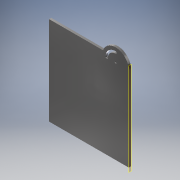
# Autodesk Inventor part: Base
Saved by Autodesk Inventor 2018 (Build 220112000, 112)
## iProperties
Created: 2021-07-05
Part Number: Base
Material: Acero, fundido
Document SubType Name: Modeling
Designer: GABRIEL
Density: 7.85 g/cm^3
Appearance: Semipulido
Author: GABRIEL
Autodesk Inventor part; units mm, degrees
ref_plane "YZ Plane" through (0, 0, 0) normal (1, 0, 0) x (0, 1, 0)
ref_plane "XZ Plane" through (0, 0, 0) normal (0, 1, 0) x (-1, 0, 0)
ref_plane "XY Plane" through (0, 0, 0) normal (0, 0, 1) x (1, 0, 0)
sketch "Boceto2" plane through (0, 0, 0) normal (0, 1, 0) x (-1, 0, 0)
  line L0 (-420, -20) -> (-420, -400)
  line L1 (-420, -400) -> (-60, -400)
  line L2 (-60, -400) -> (-60, 0)
  line L3 (-60, 0) -> (-303.4315, 0)
  arc A0 (-303.4315, 0) -> (-420, -20) centre (-360, -20) ccw
  circle A1 centre (-360, -20) radius 4
  circle A2 centre (-360, 20) radius 5
  circle A3 centre (-320, -20) radius 5
  arc A4 (-325, -20) -> (-360, 15) centre (-360, -20) ccw
  arc A5 (-315, -20) -> (-360, 25) centre (-360, -20) ccw
  dimension "d15" = 360
  dimension "d18" = 60
  dimension "d19" = 8
  dimension "d20" = 10
  dimension "d31" = 60
  dimension "d32" = 40
  dimension "d33" = 60
  dimension "d34" = 400
  dimension "d35" = 10
  dimension "d38" = 40
  constraints: 10 point on circle, 8 end point, 6 centre point, 3 coincident, 3 horizontal, 3 tangent, 1 parallel, 1 vertical
  measures "d15" distance of L1.end L0.end
  measures "d18" radius of A0
  measures "d19" diameter of A1
  measures "d20" diameter of A2
  measures "d31" distance from line of L0 A1.centre
  measures "d32" distance of A2.centre A0.centre
  measures "d33" distance from line of L0 A2.centre
  measures "d34" distance of L1.end L2.end
  measures "d35" diameter of A3
  measures "d38" horizontal distance of A2.centre A3.centre
extrude "Extrusión1" add sketch "Boceto2" along normal blind 10 contours A0 L3 L2 L1 L0 | A2 A5 A3 A4 | A3
extrude "Extrusión2" cut sketch "Boceto2" along normal blind 10 contours A2 A5 A3 A4 | A3
ref_plane "Plano de trabajo1" through (280, 0, -20) normal (1, 0, 0) x (0, 0, -1)
split body "Dividir1" result two bodies by plane through (280, 0, -20) normal (1, 0, 0) first body at (353.1726, 0.5, -274.6569)
move or copy body "Desplazar cuerpo1" bodies to move or copy 2 copy no translate (0, -50, 0)
sketch "Boceto3" plane through (420, -50, -400) normal (0, -1, 0) x (1, 0, 0)
  line L0 (-140, 400) -> (-140, 400)
  line L1 (-140, 0) -> (-140, 0)
  line L2 (-140, 0) -> (-150, 0)
  line L3 (-150, 0) -> (-150, 400)
  line L4 (-150, 400) -> (-140, 400)
  line L5 (-140, 400) -> (-140, 0)
  point P0 (-420, 400)
  dimension "d47" = 10
  dimension "d48" = 400
  constraints: 12 end point, 3 parallel, 2 horizontal, 1 perpendicular
  measures "d47" distance of L3.end L4.end
  measures "d48" distance of L2.end L3.end
extrude "Extrusión4" add sketch "Boceto3" against normal blind 50 bodies 2
